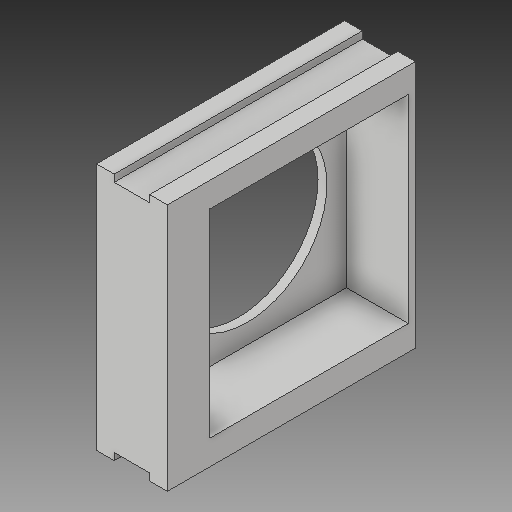
# Autodesk Inventor part: LeadScrewBox
Saved by Autodesk Inventor 2019 (Build 230136000, 136)
## iProperties
Created: 2019-06-28
Part Number: LeadScrewBox
Material: Generic
Document SubType Name: Modeling
Designer: dell
Density: 1 g/cm^3
Appearance: Default
Author: dell
Autodesk Inventor part; units mm, degrees
ref_plane "YZ Plane" through (0, 0, 0) normal (1, 0, 0) x (0, 1, 0)
ref_plane "XZ Plane" through (0, 0, 0) normal (0, 1, 0) x (-1, 0, 0)
ref_plane "XY Plane" through (0, 0, 0) normal (0, 0, 1) x (1, 0, 0)
sketch "Sketch1" plane through (0, 0, 0) normal (1, 0, 0) x (0, 1, 0)
  line L0 (-56, 56) -> (56, 56)
  line L1 (56, 56) -> (56, -56)
  line L2 (56, -56) -> (-56, -56)
  line L3 (-56, -56) -> (-56, 56)
  line L4 (-56, 56) -> (56, -56) construction
  line L5 (56, 56) -> (-56, -56) construction
  line L6 (-80, 80) -> (80, 80)
  line L7 (80, 80) -> (80, -80)
  line L8 (80, -80) -> (-80, -80)
  line L9 (-80, -80) -> (-80, 80)
  line L10 (-80, 80) -> (80, -80) construction
  line L11 (80, 80) -> (-80, -80) construction
  point P0 (0, 0)
  dimension "d0" = 112
  dimension "d1" = 112
  dimension "d2" = 160
  dimension "d3" = 160
  constraints: 24 end point, 4 midpoint, 4 parallel, 2 horizontal, 2 perpendicular
  measures "d0" distance of L1.end L2.end
  measures "d1" distance of L0.end L1.end
  measures "d2" distance of L7.end L8.end
  measures "d3" distance of L6.end L7.end
extrude "Extrusion1" add sketch "Sketch1" along normal blind 35
extrude "Extrusion2" add sketch "Sketch1" against normal blind 5 contours L0 L1 L2 L3 | L6 L7 L8 L9
sketch "Sketch2" plane through (0, 0, 0) normal (1, 0, 0) x (0, 0, -1)
  circle A0 centre (0, 0) radius 45
  dimension "d8" = 90
  constraints: 1 centre point, 1 coincident
  measures "d8" diameter of A0
extrude "Extrusion3" cut sketch "Sketch2" against normal through all
sketch "Sketch3" plane through (35, -80, 80) normal (0, 0, 1) x (1, 0, 0)
  line L0 (-35, 136) -> (-35, 24) projected
  line L1 (-35, 24) -> (0, 24) projected
  line L2 (-35, 136) -> (0, 136) projected
  line L3 (0, 0) -> (-40, 0) projected
  line L4 (-30, 0) -> (-30, 10)
  line L5 (-30, 10) -> (-10, 10)
  line L6 (-10, 10) -> (-10, 0)
  line L7 (0, 160) -> (0, 0) projected
  line L8 (-40, 0) -> (0, 0) projected
  line L9 (0, 160) -> (0, 0) projected
  line L10 (0, 160) -> (-40, 160) projected
  line L11 (-40, 0) -> (-40, 160) projected
  line L12 (-17.5, 80) -> (-40, 80)
  line L13 (-30, 0) -> (-10, 0)
  line L14 (-30, 160) -> (-30, 150)
  line L15 (-30, 150) -> (-10, 150)
  line L16 (-10, 150) -> (-10, 160)
  line L17 (-30, 160) -> (-10, 160)
  point P0 (-35, 80)
  dimension "d11" = 20
  dimension "d12" = 10
  dimension "d13" = 10
  constraints: 18 end point, 4 perpendicular, 4 symmetric about line, 2 point on line, 1 midpoint
  measures "d11" distance of L4.end L5.end
  measures "d12" distance between parallel lines of L7 L6
  measures "d13" distance of L5.end L6.end
extrude "Extrusion4" cut sketch "Sketch3" against normal through all contours L16 L15 L14 L10 | L4 L5 L6 L3
sketch "Sketch4" plane through (35, -80, -80) normal (0, 0, -1) x (-1, 0, 0)
  line L0 (0, 0) -> (0, 160) projected
  line L1 (40, 160) -> (40, 0) projected
  line L2 (0, 0) -> (40, 0)
  line L3 (40, 0) -> (40, 160)
  line L4 (40, 160) -> (0, 160)
  line L5 (0, 160) -> (0, 0)
  point P0 (35, 80)
  constraints: 8 end point, 2 parallel, 1 horizontal, 1 perpendicular
extrude "Extrusion5" cut sketch "Sketch4" against normal blind 20
sketch "Sketch5" plane through (25, -80, 80) normal (0, -1, 0) x (1, 0, 0)
  line L0 (-30, -140) -> (-30, 0) projected
  line L1 (-30, 0) -> (10, 0)
  line L2 (10, 0) -> (10, -140)
  line L3 (10, -140) -> (-30, -140)
  line L4 (-30, -140) -> (-30, 0)
  point P0 (-25, -80)
  constraints: 8 end point, 2 parallel, 1 horizontal, 1 perpendicular
extrude "Extrusion6" cut sketch "Sketch5" against normal blind 10
sketch "Sketch6" plane through (25, 80, 80) normal (0, 1, 0) x (1, 0, 0)
  line L0 (10, 0) -> (0, 0) projected
  line L1 (-30, 0) -> (-30, 140) projected
  line L2 (10, 0) -> (-30, 0)
  line L3 (-30, 0) -> (-30, 140)
  line L4 (-30, 140) -> (10, 140)
  line L5 (10, 140) -> (10, 0)
  point P0 (-25, 80)
  constraints: 8 end point, 2 parallel, 1 horizontal, 1 perpendicular
extrude "Extrusion7" cut sketch "Sketch6" against normal blind 10
sketch "Sketch7" plane through (-5, -70, 80) normal (0, -1, 0) x (1, 0, 0)
  line L0 (40, 0) -> (0, 0) projected
  line L1 (40, -140) -> (0, -140) projected
  line L2 (10, 0) -> (30, 0)
  line L3 (30, 0) -> (30, -140)
  line L4 (30, -140) -> (10, -140)
  line L5 (10, -140) -> (10, 0)
  point P0 (5, -80)
  dimension "d22" = 20
  constraints: 8 end point, 2 parallel, 2 point on line, 1 horizontal, 1 perpendicular
  measures "d22" distance of L3.end L4.end
extrude "Extrusion8" cut sketch "Sketch7" against normal blind 4
sketch "Sketch8" plane through (-5, 70, 80) normal (0, 1, 0) x (1, 0, 0)
  line L0 (30, 0) -> (40, 0) projected
  line L1 (10, 140) -> (10, 0) projected
  line L2 (30, 0) -> (10, 0)
  line L3 (10, 0) -> (10, 140)
  line L4 (10, 140) -> (30, 140)
  line L5 (30, 140) -> (30, 0)
  point P0 (5, 80)
  constraints: 8 end point, 2 parallel, 1 horizontal, 1 perpendicular
extrude "Extrusion9" cut sketch "Sketch8" against normal blind 4
body "Solid1"
